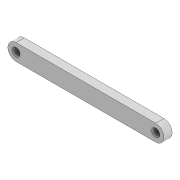
# Autodesk Inventor part: Pieza6
Saved by Autodesk Inventor 2021 (Build 250183000, 183)
## iProperties
Created: 2021-04-19
Part Number: Pieza6
Material: Genérico
Document SubType Name: Modeling
Designer: carlo
Density: 1 g/cm^3
Appearance: Valor por defecto
Mass: 4.44635 g
Surface Area: 29.427 cm^2
Volume: 4.44635 cm^3
Author: carlo
Autodesk Inventor part; units mm, degrees
ref_plane "YZ Plane" through (0, 0, 0) normal (1, 0, 0) x (0, 1, 0)
ref_plane "XZ Plane" through (0, 0, 0) normal (0, 1, 0) x (-1, 0, 0)
ref_plane "XY Plane" through (0, 0, 0) normal (0, 0, 1) x (1, 0, 0)
sketch "Boceto1" plane through (0, 0, 0) normal (0, 0, 1) x (1, 0, 0)
  arc A0 (0, 5) -> (0, -5) centre (0, 0) ccw
  arc A1 (85, -5) -> (85, 5) centre (85, 0) ccw
  line L0 (0, 5) -> (85, 5)
  line L1 (0, -5) -> (85, -5)
  circle A2 centre (0, 0) radius 2.5
  circle A3 centre (85, 0) radius 2.5
  dimension "d1" = 10
  dimension "d2" = 10
  dimension "d3" = 5
  dimension "d4" = 5
  dimension "d7" = 85
  constraints: 4 centre point, 4 end point, 4 point on circle, 3 coincident, 2 horizontal
  measures "d1" diameter of A0
  measures "d2" diameter of A1
  measures "d3" diameter of A2
  measures "d4" diameter of A3
  measures "d7" distance of A1.centre point (0, 0)
extrude "Extrusión1" add sketch "Boceto1" along normal blind 5
